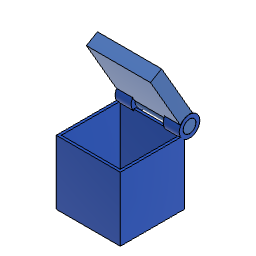
box(user parameters,joints) v1 (Autodesk Fusion 360 design; units mm, degrees)
Autodesk Fusion 360 part; units mm, degrees
sketch "Sketch1" plane through (0, 0, 0) normal (0, 0, 1) x (1, 0, 0) in component "Component"
  line L0 (0, 0) -> (50, 0)
  line L1 (50, 0) -> (50, -50)
  line L2 (50, -50) -> (0, -50)
  line L3 (0, -50) -> (0, 0)
  dimension "d5" = 50
  dimension "d6" = 50
  constraint horizontal L0
  constraint vertical L1
  constraint horizontal L2
  constraint vertical L3
  constraint coincident L0.start L3.end
  measures "d5" distance of L0.start L0.end
  measures "d6" distance of L0.end L1.end
extrude "Extrude1" add sketch "Sketch1" against normal blind 50 makes body 1 in component "Component"
shell "Shell1" thickness 2 removed faces 1 at (16.6667, -16.6667, 0) on bodies 1 in component "Component"
sketch "Sketch2" plane through (0, 0, 0) normal (1, 0, 0) x (0, 1, 0) in component "Component"
  line L0 (0, 0) -> (4, 0) construction
  line L1 (4, 0) -> (4, 4) construction
  line L2 (4, 4) -> (0, 4) construction
  line L3 (0, 4) -> (0, 0) construction
  circle A0 centre (4, 4) radius 8
  circle A1 centre (4, 4) radius 5
  circle A2 centre (4, 4) radius 4.9
  dimension "d10" = 4
  dimension "d11" = 4
  dimension "d12" = 16
  dimension "d13" = 10
  dimension "d18" = -0.1
  constraint horizontal L0
  constraint vertical L1
  constraint horizontal L2
  constraint vertical L3
  constraint coincident L0.start L3.end
  constraint coincident L1.end L2.start
  constraint concentric A0 A1
  measures "d10" distance of L1.end L2.end
  measures "d11" distance of L0.end L1.end
  measures "d12" diameter of A0
  measures "d13" diameter of A1
extrude "Extrude2" add sketch "Sketch2" along normal blind 12.5 contours A0 bodies 1 in component "Component"
move_body "Move1" bodies 1 to x (1, 0, 0) y (0, 1, 0) z (0, 0, 1) at (-50, 0, 0) in component "Component"
extrude "Extrude3" add sketch "Sketch2" against normal blind 12.5 contours A0 bodies 1 in component "Component"
extrude "Extrude4" add sketch "Sketch2" against normal blind 50 separate body contours A2 makes body 2 in component "Component"
sketch "Sketch3" plane through (0, 0, 0) normal (1, 0, 0) x (0, 1, 0) in component "Component"
  circle A0 centre (4, 4) radius 8.25
  line L0 (0, 0) -> (-50, 0)
  line L1 (-50, 0) -> (-50, 10)
  line L2 (-50, 10) -> (0, 10)
  line L3 (0, 10) -> (0, 0)
  dimension "d21" = 16.5
  dimension "d22" = 50
  dimension "d23" = 10
  constraint horizontal L0
  constraint vertical L1
  constraint horizontal L2
  constraint vertical L3
  constraint coincident L0.start L3.end
  measures "d21" diameter of A0
  measures "d22" distance of L1.end L2.end
  measures "d23" distance of L0.start L2.end
extrude "Extrude5" add sketch "Sketch3" against normal blind 50 separate body contours A0 L0 L1 L2 makes body 3 in component "Component"
extrude "Extrude6" add sketch "Sketch3" against normal blind 37.6 contours A0 L0 L2 L3 picked at (-1.2264, 5.6718) bodies 2 3 in component "Component"
extrude "Extrude9" cut sketch "Sketch3" against normal blind 12.4 contours A0 L0 L2 L3 picked at (-1.2264, 5.6718) bodies 2 in component "Component"
extrude "Extrude8" add sketch "Sketch2" against normal blind 50 contours A2 bodies 2 in component "Component"
copy_body "Body->Comp1" bodies 2 removing the originals makes body 4 in component "Component'"
copy_body "Body->Comp2" bodies 1 removing the originals makes body 5 in component "Component''"
component "Component" placed x (1, 0, 0) y (0, 1, 0) z (0, 0, 1) at (0, 0, 0)
component "Component'" placed x (1, 0, 0) y (0, 1, 0) z (0, 0, 1) at (0, 0, 0) in component "Component"
component "Component''" placed x (1, 0, 0) y (0, 1, 0) z (0, 0, 1) at (0, 0, 0) in component "Component"
equation "height = 50 mm"
equation "width = 50 mm"
equation "length = 50 mm"
equation "thickness = 2 mm"
equation "d5 = width"
equation "d6 = length"
equation "d7 = -height"
equation "d9 = thickness"
equation "d10 = thickness * 2"
equation "d11 = thickness * 2"
equation "d12 = thickness * 8"
equation "d13 = thickness * 5"
equation "d14 = width / 4"
equation "d16 = -width / 4"
equation "d19 = -width"
equation "d21 = thickness * 8 + 0.5 mm"
equation "d22 = length"
equation "d23 = thickness * 5"
equation "d24 = -width"
equation "d26 = -width * 3 / 4 - 0.1 mm"
equation "d30 = -width"
equation "d39 = -width / 4 + 0.1 mm"
